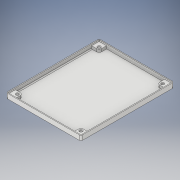
# Autodesk Inventor part: MainBoard_hf_base_sa_1
Saved by Autodesk Inventor 2019 (Build 230136000, 136)
## iProperties
Created: 2019-02-28
Part Number: MainBoard_hf_base_sa_1
Material: ABS プラスチック
Document SubType Name: Modeling
Designer: shun
Density: 1.06 g/cm^3
Appearance: 滑らか - 白
Author: shun
Autodesk Inventor part; units mm, degrees
ref_plane "YZ Plane" through (0, 0, 0) normal (1, 0, 0) x (0, 1, 0)
ref_plane "XZ Plane" through (0, 0, 0) normal (0, 1, 0) x (-1, 0, 0)
ref_plane "XY Plane" through (0, 0, 0) normal (0, 0, 1) x (1, 0, 0)
sketch "スケッチ1" plane through (0, 0, 0) normal (0, 1, 0) x (-1, 0, 0)
  line L0 (40, 50) -> (-40, 50) construction
  line L1 (-40, 50) -> (-40, -50) construction
  line L2 (-40, -50) -> (40, -50) construction
  line L3 (40, -50) -> (40, 50) construction
  line L4 (40, 50) -> (-40, -50) construction
  line L5 (-40, 50) -> (40, -50) construction
  line L6 (40.3, 50.3) -> (-40.3, 50.3)
  line L7 (-40.3, 50.3) -> (-40.3, -50.3)
  line L8 (-40.3, -50.3) -> (40.3, -50.3)
  line L9 (40.3, -50.3) -> (40.3, 50.3)
  line L10 (41.3, 51.3) -> (-41.3, 51.3)
  line L11 (-41.3, 51.3) -> (-41.3, -51.3)
  line L12 (-41.3, -51.3) -> (41.3, -51.3)
  line L13 (41.3, -51.3) -> (41.3, 51.3)
  line L14 (-35, 45) -> (35, 45) construction
  line L15 (35, 45) -> (35, -45) construction
  line L16 (35, -45) -> (-35, -45) construction
  line L17 (-35, -45) -> (-35, 45) construction
  line L18 (32, 50.3) -> (32, 45)
  arc A0 (32, 45) -> (35, 42) centre (35, 45) ccw
  line L19 (35, 42) -> (40.3, 42)
  line L20 (0, 0) -> (0, 50.3)
  line L21 (0, 50.3) -> (0, 51.3)
  line L22 (0, 0) -> (40.3, 0)
  line L23 (40.3, 0) -> (41.3, 0)
  dimension "d0" = 80
  dimension "d1" = 100
  dimension "d2" = 0.3
  dimension "d3" = 1
  dimension "d4" = 5
  dimension "d5" = 3
  constraints: 48 end point, 8 parallel, 6 midpoint, 6 perpendicular, 5 coincident, 4 point on line, 2 point on circle, 1 centre point, 1 horizontal, 9 other
  measures "d0" distance of L2.end L1.end
  measures "d1" distance of L1.end L0.end
  measures "d2" distance between parallel lines of L3 L9
  measures "d3" distance between parallel lines of L9 L13
  measures "d4" distance between parallel lines of L0 L14
  measures "d5" distance from line of L18 point (35, 45)
extrude "押し出し1" add sketch "スケッチ1" against normal blind 0.7 contours L9 L19 A0 L18 L6 | L6 L21 L10 L13 L23 L9 | L18 A0 L19 L9 L22 L20 L6
extrude "押し出し2" add sketch "スケッチ1" along normal blind 3 contours L9 L19 A0 L18 L6
extrude "押し出し3" add sketch "スケッチ1" along normal blind 1.5 and the other way blind 3 from surface at 3 contours L6 L21 L10 L13 L23 L9
hole "穴1" at (35, 0, 45) at (-35, 0, 45) at (-35, 0, -45) at (35, 0, -45) direction (0, -1, 0) diameter 2.5 end through all both
fillet "フィレット1" radius 0.5 1 edges at (-35, 3, 43.75)
mirror "ミラー1" about plane through (-41.3, 0, 0) normal (0, 0, -1) of "フィレット1", "穴1", "押し出し3", "押し出し2", "押し出し1"
mirror "ミラー2" about plane through (0, 0, 50.3) normal (1, 0, 0) of "フィレット1", "穴1", "押し出し3", "押し出し2", "押し出し1", "ミラー1"
fillet "フィレット2" radius 1 2 edges at (-40.3, 0, 0) (0, 0, 50.3)
fillet "フィレット3" radius 2 4 edges at (41.3, 1.9, 51.3) (-41.3, 1.9, 51.3) (-41.3, 1.9, -51.3) (41.3, 1.9, -51.3)
